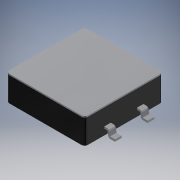
# Autodesk Inventor part: TACT-SWITCH-SMD-12X12MM
Saved by Autodesk Inventor 2018.3 (Build 223284000, 284)
## iProperties
Created: 2020-10-19
Part Number: TACT-SWITCH-SMD-12X12MM
Material: Genérico
Document SubType Name: Modeling
Designer: laguerre
Density: 8.47 g/cm^3
Appearance: Suave - Negro
Author: laguerre
Autodesk Inventor part; units mm, degrees
ref_plane "YZ Plane" through (0, 0, 0) normal (1, 0, 0) x (0, 1, 0)
ref_plane "XZ Plane" through (0, 0, 0) normal (0, 1, 0) x (-1, 0, 0)
ref_plane "XY Plane" through (0, 0, 0) normal (0, 0, 1) x (1, 0, 0)
sketch "Boceto39" plane through (0, 0, 0) normal (0, 0, 1) x (1, 0, 0)
  line L0 (-5.5, 6) -> (5.5, 6)
  line L1 (6, 5.5) -> (6, -5.5)
  line L2 (5.5, -6) -> (-5.5, -6)
  line L3 (-6, -5.5) -> (-6, 5.5)
  arc A0 (6, 5.5) -> (5.5, 6) centre (5.5, 5.5) ccw
  arc A1 (-5.5, 6) -> (-6, 5.5) centre (-5.5, 5.5) ccw
  arc A2 (-6, -5.5) -> (-5.5, -6) centre (-5.5, -5.5) ccw
  arc A3 (5.5, -6) -> (6, -5.5) centre (5.5, -5.5) ccw
  point P0 (0, 0)
  point P1 (-6, 6)
  point P2 (6, -6)
  point P3 (6, 6)
  point P4 (-6, -6)
  point P5 (0, 6)
  point P6 (6, 0)
  dimension "d373" = 12
  dimension "d376" = 0.5
  constraints: 8 end point, 8 point on circle, 8 point on line, 8 tangent, 4 centre point, 3 equal radius, 2 midpoint, 2 parallel, 2 perpendicular, 1 horizontal, 1 horizontal alignment, 1 vertical alignment
  measures "d373" distance of point (-6, 6) point (6, 6)
  measures "d376" radius of A0
extrude "Extrusión13" add sketch "Boceto39" along normal blind 3.7
sketch "Boceto40" plane through (0, 0, 3.7) normal (0, 0, 1) x (1, 0, 0)
  line L0 (5.5, 6) -> (-5.5, 6) projected
  arc A0 (-5.5, 6) -> (-6, 5.5) centre (-5.5, 5.5) ccw projected
  line L1 (-6, 5.5) -> (-6, -5.5) projected
  arc A1 (-6, -5.5) -> (-5.5, -6) centre (-5.5, -5.5) ccw projected
  line L2 (-5.5, -6) -> (5.5, -6) projected
  arc A2 (5.5, -6) -> (6, -5.5) centre (5.5, -5.5) ccw projected
  line L3 (6, -5.5) -> (6, 5.5) projected
  arc A3 (6, 5.5) -> (5.5, 6) centre (5.5, 5.5) ccw projected
  point P0 (0, 0)
extrude "Extrusión14" add sketch "Boceto40" along normal blind 0.2 separate body
sketch "Boceto43" plane through (0, 0, 0) normal (1, 0, 0) x (0, 1, 0)
  line L0 (0, 0) -> (0, -3.6276) construction
  line L1 (6, 0) -> (6, 3.7) construction
  line L2 (6.4016, 1.2) -> (6, 1.2)
  line L3 (5.5, 3.9) -> (-5.5, 3.9) projected
  line L4 (5.5, 0) -> (-5.5, 0) projected
  line L5 (6.4016, 0.9) -> (6, 0.9)
  line L6 (6, 0.9) -> (6, 1.2)
  arc A0 (6.5, 0.818) -> (6.4016, 0.9) centre (6.4016, 0.8) ccw
  arc A1 (6.7951, 0.8721) -> (6.4016, 1.2) centre (6.4016, 0.8) ccw
  line L7 (6.7951, 0.8721) -> (6.885, 0.382)
  line L8 (6.9833, 0.3) -> (7.65, 0.3)
  line L9 (7.65, 0.3) -> (7.65, 0)
  line L10 (7.65, 0) -> (6.9833, 0)
  line L11 (6.5899, 0.3279) -> (6.5, 0.818)
  arc A2 (6.885, 0.382) -> (6.9833, 0.3) centre (6.9833, 0.4) ccw
  arc A3 (6.5899, 0.3279) -> (6.9833, 0) centre (6.9833, 0.4) ccw
  point P0 (6.55, 1.2)
  point P1 (6.65, 0)
  dimension "d399" = 2.7
  dimension "d426" = 0.3
  dimension "d435" = 0.1
  dimension "d436" = 0.4
  dimension "d437" = 0.3
  dimension "d438" = 0.3
  dimension "d439" = 7.65
  dimension "d440" = 6.5
  dimension "d441" = 1
  dimension "d442" = 0.1
  dimension "d443" = 0.4
  constraints: 18 end point, 8 point on circle, 8 tangent, 5 point on line, 4 centre point, 3 perpendicular, 2 collinear, 1 horizontal, 1 parallel, 1 vertical
  measures "d399" distance between parallel lines of L2 L3
  measures "d426" distance between parallel lines of L2 L5
  measures "d435" radius of A0
  measures "d436" radius of A1
  measures "d437" distance between parallel lines of L8 L10
  measures "d438" distance between parallel lines of L11 L7
  measures "d439" distance between parallel lines of L0 L9
  measures "d440" distance from line of L0 L11.end
  measures "d441" distance of L9.end point (6.65, 0)
  measures "d442" radius of A2
  measures "d443" radius of A3
extrude "Extrusión15" add sketch "Boceto43" along normal mid plane 6 separate body
sketch "Boceto45" plane through (0, 0, 0) normal (1, 0, 0) x (0, 1, 0)
  line L0 (6, 1.2) -> (6.4016, 1.2) projected
  line L1 (6, 1.2) -> (8.6614, 1.2)
  line L2 (8.6614, 1.2) -> (8.6614, -2.2134)
  line L3 (8.6614, -2.2134) -> (6, -2.2134)
  line L4 (6, -2.2134) -> (6, 1.2)
  point P0 (0, 0)
  point P1 (3.3, 0.8)
  constraints: 8 end point, 2 parallel, 1 horizontal, 1 perpendicular, 1 other
extrude "Extrusión17" cut sketch "Boceto45" along normal mid plane 4 bodies 3
sketch "Boceto46" plane through (0, 0, 3.9) normal (0, 0, 1) x (1, 0, 0)
  line L0 (-5, -5) -> (5, -5) construction
  line L1 (5, -5) -> (5, 5) construction
  line L2 (5, 5) -> (-5, 5) construction
  line L3 (-5, 5) -> (-5, -5) construction
  circle A0 centre (-5, -5) radius 0.5
  circle A1 centre (-5, 5) radius 0.5
  circle A2 centre (5, 5) radius 0.5
  circle A3 centre (5, -5) radius 0.5
  point P0 (0, 0)
  point P1 (0, -5)
  point P2 (-5, 0)
  dimension "d417" = 1
  dimension "d418" = 10
  constraints: 8 end point, 4 centre point, 4 coincident, 3 equal radius, 2 midpoint, 2 parallel, 2 perpendicular, 1 horizontal, 1 horizontal alignment, 1 vertical alignment
  measures "d417" diameter of A0
  measures "d418" distance of L1.end L2.end
sketch "Boceto48" plane through (0, 0, 0) normal (0, 1, 0) x (-1, 0, 0)
  line L0 (0, 0) -> (0, 17.1627)
  line L1 (-5.5, 3.9) -> (5.5, 3.9) construction
  line L2 (0, 3.9) -> (-3.35, 3.9)
  line L3 (-3.35, 3.9) -> (-3.343, 4.3)
  line L4 (-3.343, 4.3) -> (0, 4.3)
  line L5 (0, 4.3) -> (0, 3.9)
  line L6 (-5.5, 0) -> (5.5, 0) projected
  line L7 (-3.35, 3.9) -> (-3.35, 4.5675) construction
  dimension "d422" = 4.3
  dimension "d423" = 6.7
  dimension "d424" = 1
  constraints: 12 end point, 2 perpendicular, 2 point on line, 2 vertical, 1 midpoint
  measures "d422" distance between parallel lines of L6 L4
  measures "d423" diameter of L2.end L0
  measures "d424" angle of L7 L3
